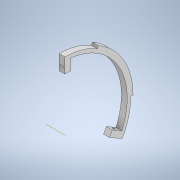
# Autodesk Inventor part: new_insert
Saved by Autodesk Inventor 2021 (Build 250183000, 183)
## iProperties
Created: 2020-09-16
Part Number: new_insert
Material: Generic
Document SubType Name: Modeling
Designer: dsouthall
Density: 1 g/cm^3
Appearance: Default
Author: dsouthall
Autodesk Inventor part; units mm, degrees
ref_plane "YZ Plane" through (0, 0, 0) normal (1, 0, 0) x (0, 1, 0)
ref_plane "XZ Plane" through (0, 0, 0) normal (0, 1, 0) x (-1, 0, 0)
ref_plane "XY Plane" through (0, 0, 0) normal (0, 0, 1) x (1, 0, 0)
sketch "Part" plane through (0, 0, 0) normal (1, 0, 0) x (0, 1, 0)
  line L0 (-0.5368, 0.0583) -> (59.7882, 0.0583) construction
  line L1 (-0.5371, -0.7417) -> (44.8022, -0.7417) construction
  arc A0 (59.7829, -0.7417) -> (59.7882, 0.0583) centre (-0.5368, 0.0583) ccw construction
  line L2 (-0.5368, 0.0583) -> (49.9741, -29.1042) construction
  arc A1 (47.3067, -27.5642) -> (54.7024, -0.7417) centre (-0.5368, 0.0583) ccw construction
  line L3 (69.9104, -5.8217) -> (54.3944, -5.8217) construction
  arc A2 (51.7936, -29.9522) -> (59.7829, -0.7417) centre (-0.5368, 0.0583) ccw construction
  line L4 (-0.5368, 0.0583) -> (66.9803, -116.8847) construction
  arc A3 (29.6257, -52.1846) -> (51.7936, -29.9522) centre (-0.5368, 0.0583) ccw
  arc A4 (27.0857, -47.7852) -> (54.3944, -5.8217) centre (-0.5368, 0.0583) ccw
  arc A5 (54.7024, -0.7417) -> (54.7082, 0.0583) centre (-0.5368, 0.0583) ccw construction
  line L5 (54.7024, -0.7417) -> (59.7829, -0.7417) construction
  line L6 (57.491, -5.8217) -> (54.3944, -5.8217) construction
  line L7 (44.8022, 0.0583) -> (44.8022, -0.7417) construction
  line L8 (44.8022, -0.7417) -> (44.8022, -5.8217)
  line L9 (44.8022, -5.8217) -> (44.8022, -11.0315) construction
  line L10 (44.8022, -0.7417) -> (57.7827, -0.7417)
  line L11 (44.8022, -5.8217) -> (-19.8971, -5.8217) construction
  line L12 (49.2882, 5.599) -> (49.2882, -56.7812) construction
  arc A6 (28.6257, -50.4526) -> (49.9741, -29.1042) centre (-0.5368, 0.0583) ccw construction
  line L13 (54.3944, -5.8217) -> (50.4651, -5.8217) construction
  line L14 (54.3944, -5.8217) -> (44.8022, -5.8217)
  line L15 (49.9741, -29.1042) -> (51.7936, -29.9522)
  arc A7 (49.9741, -29.1042) -> (57.7827, -0.7417) centre (-0.5368, 0.0583) ccw
  arc A8 (57.7827, -0.7417) -> (57.7882, 0.0583) centre (-0.5368, 0.0583) ccw construction
  line L16 (-0.5368, 0.0583) -> (-30.6993, -52.1846) construction
  line L17 (0.1561, -0.3414) -> (-22.5135, -39.6064) construction
  arc A9 (-30.6993, -52.1846) -> (-30.0039, -52.5801) centre (-0.5368, 0.0583) ccw construction
  line L18 (-0.5368, 0.0583) -> (-0.5368, -58.2667) construction
  arc A10 (-27.4636, -48.1802) -> (-0.5368, -55.1867) centre (-0.5368, 0.0583) ccw construction
  line L19 (-30.6682, -63.8907) -> (-22.9102, -50.4535) construction
  arc A11 (-30.0039, -52.5801) -> (-0.7122, -60.2664) centre (-0.5368, 0.0583) ccw construction
  arc A12 (-0.7122, -60.2664) -> (29.6257, -52.1846) centre (-0.5368, 0.0583) ccw
  arc A13 (-22.9102, -50.4535) -> (27.0857, -47.7852) centre (-0.5368, 0.0583) ccw
  arc A14 (-28.1593, -47.7852) -> (-27.4636, -48.1802) centre (-0.5368, 0.0583) ccw construction
  line L20 (-27.4636, -48.1802) -> (-30.0039, -52.5801) construction
  line L21 (-24.4585, -53.1353) -> (-22.9102, -50.4535) construction
  line L22 (-23.2063, -39.2064) -> (-22.5135, -39.6064) construction
  line L23 (-22.5135, -39.6064) -> (-18.1141, -42.1464)
  line L24 (-18.1141, -42.1464) -> (-13.6022, -44.7513) construction
  line L25 (-22.5135, -39.6064) -> (-29.0038, -50.8478)
  line L26 (-18.1141, -42.1464) -> (14.2355, 13.8848) construction
  line L27 (-30.2477, -40.3211) -> (23.7751, -71.5111) construction
  arc A15 (-0.5368, -58.2667) -> (28.6257, -50.4526) centre (-0.5368, 0.0583) ccw construction
  line L28 (-22.9102, -50.4535) -> (-20.9456, -47.0506) construction
  line L29 (-22.9102, -50.4535) -> (-18.1141, -42.1464)
  line L30 (-0.5368, -58.2667) -> (-0.7122, -60.2664)
  arc A16 (-29.0038, -50.8478) -> (-0.5368, -58.2667) centre (-0.5368, 0.0583) ccw
  arc A17 (-29.6993, -50.4526) -> (-29.0038, -50.8478) centre (-0.5368, 0.0583) ccw construction
  dimension "d29" = 60.325
  dimension "d32" = 30
  dimension "d35" = 5.08
  dimension "d37" = 60
  dimension "d38" = 55.245
  dimension "d42" = 14.986
  dimension "d44" = 10.5
  dimension "d45" = 58.325
  dimension "d64" = 0.8
  constraints: 62 end point, 46 point on circle, 21 symmetric about line, 19 point on line, 18 centre point, 18 parallel, 10 coincident, 4 perpendicular, 1 horizontal, 9 other
  measures "d29" distance of L0.start L0.end
  measures "d32" angle of L1 L2
  measures "d35" distance between parallel lines of L1 L3
  measures "d37" angle of L4 L0
  measures "d38" radius of A1
  measures "d42" distance of L0.end L7.start
  measures "d44" distance from line of L12 L0.end
  measures "d45" radius of A6
  measures "d64" distance between parallel lines of L0 L1
extrude "Extrusion2" add sketch "Part" along normal blind 5.08
sketch "Sketch5" plane through (0, 44.8022, -0.7417) normal (0, 0, 1) x (1, 0, 0)
  line L0 (0, 12.9805) -> (5.08, 12.9805) projected
  line L1 (2.54, 12.9805) -> (2.54, 0) construction
  line L2 (0, 0) -> (5.08, 0) projected
  line L3 (0, 4.4805) -> (5.08, 4.4805) construction
  point P0 (0, -44.8022)
  point P1 (2.54, 4.4805)
  dimension "d48" = 8.5
  constraints: 4 end point, 3 midpoint, 1 horizontal
  measures "d48" distance between parallel lines of L0 L3
hole "Hole1" at (2.54, 49.2827, -0.7417) direction (0, 0, -1) diameter 2.4384 depth 12.2936 tip angle 118 clearance for "Flat Head Machine Screw (82)" size "#2" standard "Ansi Unified Screw Threads"
sketch "Sketch6" plane through (0, -29.0038, -50.8478) normal (0, -0.866, 0.5) x (1, 0, 0)
  line L0 (0, 12.9805) -> (5.08, 12.9805) construction
  line L1 (2.54, 12.9805) -> (2.54, 0) construction
  line L2 (0, 0) -> (5.08, 0) construction
  line L3 (0, 5.9891) -> (0, 58.4948) construction
  line L4 (0, 8.5) -> (5.08, 8.5) construction
  line L5 (5.08, 5.9891) -> (5.08, 58.4948) construction
  point P0 (0, 58.5374)
  point P1 (2.54, 8.5)
  dimension "d56" = 8.5
  constraints: 4 end point, 3 midpoint, 2 point on line, 1 perpendicular
  measures "d56" distance between parallel lines of L2 L4
hole "Hole2" at (2.54, -24.7538, -43.4866) direction (0, 0.866, -0.5) diameter 2.4384 depth 12.2936 tip angle 118 clearance for "Flat Head Machine Screw (82)" size "#2" standard "Ansi Unified Screw Threads"
equation "\"d35\" = d29 - d34"
equation "\"d34\" = 55.245"
body "Solid2"
